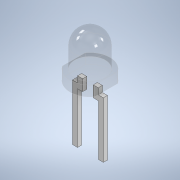
# Autodesk Inventor part: TEFT4300
Saved by Autodesk Inventor 2021 (Build 250183000, 183)
## iProperties
Created: 2021-06-29
Part Number: TEFT4300
Material: Generic
Document SubType Name: Modeling
Designer: ermoz
Density: 1 g/cm^3
Appearance: Default
Author: ermoz
Autodesk Inventor part; units mm, degrees
ref_plane "YZ Plane" through (0, 0, 0) normal (1, 0, 0) x (0, 1, 0)
ref_plane "XZ Plane" through (0, 0, 0) normal (0, 1, 0) x (-1, 0, 0)
ref_plane "XY Plane" through (0, 0, 0) normal (0, 0, 1) x (1, 0, 0)
sketch "Sketch1" plane through (0, 0, 0) normal (1, 0, 0) x (0, 1, 0)
  arc A0 (1.5, 0) -> (0, 1.5) centre (0, 0) ccw
  line L0 (-3, 0) -> (-3, 1.5)
  line L1 (-3, 1.5) -> (0, 1.5)
  line L2 (1.5, 0) -> (-3, 0)
  dimension "d0" = 1.5
  dimension "d1" = 4.5
  constraints: 6 end point, 3 point on circle, 1 centre point, 1 coincident, 1 parallel, 1 perpendicular, 1 vertical
  measures "d0" radius of A0
  measures "d1" distance from line of L0 L2.start
revolve "Revolution1" add sketch "Sketch1" angle 360 about axis through (0, 1.5, 0) along (0, -1, 0)
sketch "Sketch2" plane through (0, -3, 0) normal (0, -1, 0) x (1, 0, 0)
  circle A0 centre (0, 0) radius 1.95
  dimension "d3" = 3.9
  constraints: 1 centre point, 1 coincident
  measures "d3" diameter of A0
extrude "Extrusion1" add sketch "Sketch2" against normal blind 1
sketch "Sketch3" plane through (0, -3, 0) normal (0, -1, 0) x (1, 0, 0)
  circle A0 centre (0, 0) radius 1.6
  line L0 (1.6, -1.1147) -> (1.6, 1.1147)
  line L1 (-1.6, -1.1147) -> (-1.6, 1.1147)
  circle A1 centre (0, 0) radius 1.95 projected
  dimension "d6" = 3.2
  constraints: 4 end point, 4 point on circle, 2 tangent, 2 vertical, 1 centre point, 1 coincident
  measures "d6" diameter of A0
extrude "Extrusion2" cut sketch "Sketch3" against normal through all contours L0 A1 | L1 A1
sketch "Sketch4" plane through (0, -3, 0) normal (0, -1, 0) x (1, 0, 0)
  line L0 (1.02, -0.2) -> (0.52, -0.2)
  line L1 (0.52, -0.2) -> (0.52, 0.2)
  line L2 (0.52, 0.2) -> (1.02, 0.2)
  line L3 (1.02, 0.2) -> (1.02, -0.2)
  line L4 (1.02, -0.2) -> (0.52, 0.2) construction
  line L5 (0.52, -0.2) -> (1.02, 0.2) construction
  line L6 (-0.52, -0.2) -> (-1.02, -0.2)
  line L7 (-1.02, -0.2) -> (-1.02, 0.2)
  line L8 (-1.02, 0.2) -> (-0.52, 0.2)
  line L9 (-0.52, 0.2) -> (-0.52, -0.2)
  line L10 (-0.52, -0.2) -> (-1.02, 0.2) construction
  line L11 (-1.02, -0.2) -> (-0.52, 0.2) construction
  line L12 (0, 0) -> (0, -0.871)
  line L13 (0, 0) -> (-0.6551, 0)
  point P0 (0.77, 0)
  point P1 (-0.77, 0)
  point P2 (-0.77, 0)
  point P3 (0.77, 0)
  point P4 (-0.77, 0)
  dimension "d9" = 1.54
  dimension "d10" = 0.4
  dimension "d11" = 0.5
  constraints: 28 end point, 7 midpoint, 4 parallel, 3 horizontal, 2 equal length, 2 perpendicular, 1 horizontal alignment, 1 point on line, 1 vertical, 1 other
  measures "d9" distance of point (0.77, 0) point (-0.77, 0)
  measures "d10" distance of L6.end L7.end
  measures "d11" distance of L7.end L8.end
extrude "Extrusion3" add sketch "Sketch4" along normal blind 1.1 separate body
sketch "Sketch5" plane through (0, -4.1, 0) normal (0, -1, 0) x (1, 0, 0)
  line L0 (0.52, -0.2) -> (1.02, -0.2) projected
  line L1 (0.52, -0.2) -> (1.52, -0.2)
  line L2 (1.52, -0.2) -> (1.52, 0.2)
  line L3 (1.52, 0.2) -> (0.52, 0.2)
  line L4 (0.52, 0.2) -> (0.52, -0.2)
  line L5 (-0.52, -0.2) -> (-0.52, 0.2) projected
  line L6 (-0.52, -0.2) -> (-1.52, -0.2)
  line L7 (-1.52, -0.2) -> (-1.52, 0.2)
  line L8 (-1.52, 0.2) -> (-0.52, 0.2)
  line L9 (-0.52, 0.2) -> (-0.52, -0.2)
  line L10 (1.02, -0.2) -> (1.52, -0.2)
  line L11 (1.52, -0.2) -> (1.52, 0.2)
  line L12 (1.52, 0.2) -> (1.02, 0.2)
  line L13 (1.02, 0.2) -> (1.02, -0.2)
  line L14 (-1.02, -0.2) -> (-0.52, -0.2) projected
  line L15 (-1.02, 0.2) -> (-1.02, -0.2) projected
  line L16 (-0.52, -0.2) -> (-1.02, -0.2)
  line L17 (-1.02, -0.2) -> (-1.02, 0.2)
  line L18 (-1.02, 0.2) -> (-0.52, 0.2)
  line L19 (-0.52, 0.2) -> (-0.52, -0.2)
  point P0 (0, 0)
  dimension "d14" = 1
  dimension "d15" = 1
  constraints: 32 end point, 8 parallel, 4 horizontal, 4 perpendicular, 1 point on line
  measures "d14" distance of L3.end L2.end
  measures "d15" distance of L7.end L8.end
extrude "Extrusion4" add sketch "Sketch5" along normal blind 5 and the other way blind 0.5 contours L13 L3 L2 L1 | L6 L7 L8 L15 bodies 2
body "Solid1"
body "Solid2"
